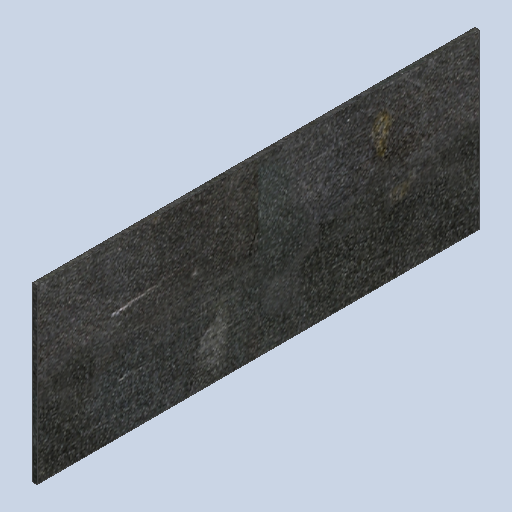
# Autodesk Inventor part: AI-Cover
Saved by Autodesk Inventor 2024.3 (Build 283343000, 343)
## iProperties
Created: 2025-06-26
Part Number: AI-Cover
Material: Steel
Document SubType Name: Sheet Metal
Designer: ajclo
Density: 7.85 g/cm^3
Sheet Metal Rule: Default_mm
Appearance: Plate
Mass: 244.92 g
Surface Area: 323.12 cm^2
Volume: 31.2 cm^3
Author: ajclo
Autodesk Inventor part; units mm, degrees
ref_plane "YZ Plane" through (0, 0, 0) normal (1, 0, 0) x (0, 1, 0)
ref_plane "XZ Plane" through (0, 0, 0) normal (0, 1, 0) x (-1, 0, 0)
ref_plane "XY Plane" through (0, 0, 0) normal (0, 0, 1) x (1, 0, 0)
sketch "Sketch1" plane through (0, 0, 0) normal (1, 0, 0) x (0, 1, 0)
  line L0 (-39, 100) -> (39, 100)
  line L1 (39, 100) -> (39, -100)
  line L2 (39, -100) -> (-39, -100)
  line L3 (-39, -100) -> (-39, 100)
  line L4 (-39, 100) -> (39, -100) construction
  line L5 (39, 100) -> (-39, -100) construction
  line L6 (39, 100) -> (30, 100)
  line L7 (39, -100) -> (30, -100)
  point P0 (0, 0)
  point P1 (0, 0)
  dimension "d0" = 200
  dimension "d6" = 78
  measures "d0" distance of L0.end L1.end
  measures "d6" distance of L1.end L2.end
extrude "Plate1" add sketch "Sketch1" along normal blind 2
equation "\"d5\" = Thickness"
equation "\"BendRadius\" = Thickness"
equation "\"BendReliefWidth\" = Thickness"
equation "\"BendReliefDepth\" = 0.5 * Thickness"
equation "\"CornerReliefSize\" = 4 * Thickness"
equation "\"MinimumRemnant\" = 2 * Thickness"
equation "\"TransitionRadius\" = BendRadius"
equation "\"JacobiRadiusSize\" = BendRadius"
equation "\"GapSize\" = Thickness"
equation "\"Thickness\" = 2"
body "Solid1"
